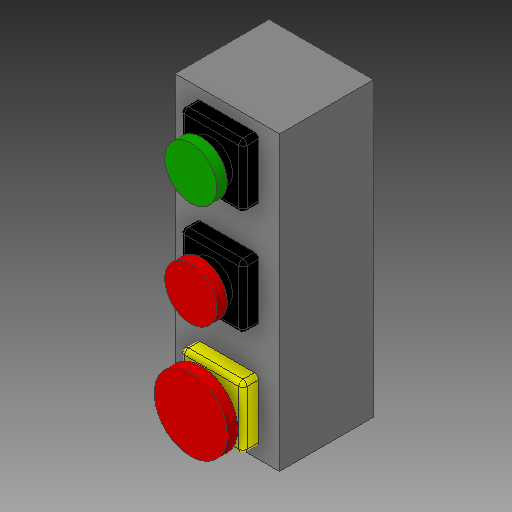
# Autodesk Inventor part: Botones
Saved by Autodesk Inventor 2019 (Build 230136000, 136)
## iProperties
Created: 2019-08-01
Part Number: Botones
Material: Generic
Document SubType Name: Modeling
Designer: felix
Density: 1 g/cm^3
Appearance: Default
Mass: 2794.49 g
Surface Area: 1507.91 cm^2
Volume: 2794.49 cm^3
Author: felix
Autodesk Inventor part; units mm, degrees
ref_plane "YZ Plane" through (0, 0, 0) normal (1, 0, 0) x (0, 1, 0)
ref_plane "XZ Plane" through (0, 0, 0) normal (0, 1, 0) x (-1, 0, 0)
ref_plane "XY Plane" through (0, 0, 0) normal (0, 0, 1) x (1, 0, 0)
sketch "Sketch1" plane through (0, 0, 0) normal (0, 0, 1) x (1, 0, 0)
  line L0 (0, 280) -> (100, 280)
  line L1 (100, 280) -> (100, 0)
  line L2 (100, 0) -> (0, 0)
  line L3 (0, 0) -> (0, 280)
  dimension "d0" = 280
  dimension "d1" = 100
  constraints: 8 end point, 2 parallel, 1 coincident, 1 horizontal, 1 perpendicular
  measures "d0" distance of L0.end L1.end
  measures "d1" distance of L0.start L0.end
extrude "Extrusion1" add sketch "Sketch1" along normal blind 90
sketch "Sketch2" plane through (0, 0, 90) normal (0, 0, 1) x (1, 0, 0)
  line L0 (20, 270) -> (80, 270)
  line L1 (80, 270) -> (80, 210)
  line L2 (80, 210) -> (20, 210)
  line L3 (20, 210) -> (20, 270)
  line L4 (20, 170) -> (80, 170)
  line L5 (80, 170) -> (80, 110)
  line L6 (80, 110) -> (20, 110)
  line L7 (20, 110) -> (20, 170)
  line L8 (20, 70) -> (80, 70)
  line L9 (80, 70) -> (80, 10)
  line L10 (80, 10) -> (20, 10)
  line L11 (20, 10) -> (20, 70)
  point P0 (0, 0)
  dimension "d4" = 20
  dimension "d5" = 80
  dimension "d6" = 270
  dimension "d7" = 210
  dimension "d8" = 10
  dimension "d9" = 70
  dimension "d10" = 110
  dimension "d11" = 170
  constraints: 24 end point, 7 parallel, 3 horizontal, 3 perpendicular, 3 point on line
  measures "d4" distance from line of point (0, 0) L3
  measures "d5" distance from line of point (0, 0) L1
  measures "d6" distance from line of point (0, 0) L0
  measures "d7" distance from line of point (0, 0) L2
  measures "d8" distance from line of point (0, 0) L10
  measures "d9" distance from line of point (0, 0) L8
  measures "d10" distance from line of point (0, 0) L6
  measures "d11" distance from line of point (0, 0) L4
extrude "Extrusion2" add sketch "Sketch2" along normal blind 15
fillet "Fillet1" radius 4 12 edges at (80, 270, 97.5) (80, 170, 97.5) (80, 70, 97.5) (80, 210, 97.5) (80, 110, 97.5) (80, 10, 97.5) (20, 270, 97.5) (20, 210, 97.5) (20, 170, 97.5) (20, 110, 97.5) (20, 70, 97.5) (20, 10, 97.5)
fillet "Fillet2" radius 4 24 edges at (78.8284, 268.8284, 105) (50, 270, 105) (21.1716, 268.8284, 105) (20, 240, 105) (21.1716, 211.1716, 105) (50, 210, 105) (78.8284, 211.1716, 105) (80, 240, 105) (21.1716, 168.8284, 105) (20, 140, 105) (21.1716, 111.1716, 105) (50, 110, 105) (78.8284, 111.1716, 105) (80, 140, 105) (78.8284, 168.8284, 105) (50, 170, 105) (21.1716, 68.8284, 105) (20, 40, 105) (21.1716, 11.1716, 105) (50, 10, 105) (78.8284, 11.1716, 105) (80, 40, 105) (78.8284, 68.8284, 105) (50, 70, 105)
sketch "Sketch3" plane through (0, 0, 105) normal (0, 0, 1) x (1, 0, 0)
  circle A0 centre (50, 240) radius 20
  line L0 (0, 336) -> (0, -56) projected
  circle A1 centre (50, 140) radius 20
  circle A2 centre (50, 40) radius 20
  point P0 (0, 0)
  dimension "d16" = 240
  dimension "d17" = 40
  dimension "d18" = 50
  dimension "d21" = 100
  constraints: 3 centre point, 1 vertical, 4 other
  measures "d16" vertical distance of point (0, 0) A0.centre
  measures "d17" diameter of A0
  measures "d18" horizontal distance of point (0, 0) A0.centre
  measures "d21" distance of A0.centre A1.centre
extrude "Extrusion3" add sketch "Sketch3" along normal blind 10
sketch "Sketch4" plane through (50, 240, 115) normal (0, 0, 1) x (1, 0, 0)
  circle A0 centre (0, 0) radius 20 projected
  circle A1 centre (0, 0) radius 25
  line L0 (-50, 96) -> (-50, -296) projected
  circle A2 centre (0, -100) radius 25
  circle A3 centre (0, -200) radius 35
  point P0 (-50, -240)
  dimension "d28" = 50
  dimension "d31" = 100
  dimension "d36" = 200
  dimension "d37" = 70
  constraints: 3 centre point, 1 coincident, 1 vertical, 1 vertical alignment, 2 other
  measures "d28" diameter of A1
  measures "d31" distance of A1.centre A2.centre
  measures "d36" distance of A1.centre A3.centre
  measures "d37" diameter of A3
extrude "Extrusion4" add sketch "Sketch4" along normal blind 10 contours A0 | A1 | A2 | A3
body "Solid1"
